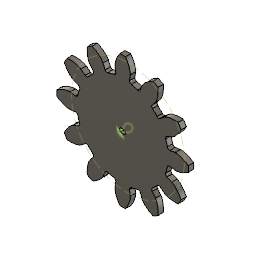
new wheel (Autodesk Fusion 360 design; units mm, degrees)
description: Spur Gear; Module: 8.7; Num Teeth: 12; Pressure Angle: 20.0; Backlash: 0.00 mm
part number: 2026-03-19-09-10-25-841
Autodesk Fusion 360 part; units mm, degrees
sketch "Base Circle" plane through (0, 0, 0) normal (0, 0, 1) x (1, 0, 0)
  circle A0 centre (0, 0) radius 42.1341
  circle A1 centre (0, 0) radius 2.7
extrude "Extrude1" add sketch "Base Circle" along normal blind 10
sketch "Gear Tooth" plane through (0, 0, 0) normal (0, 0, 1) x (1, 0, 0)
  spline S0 degree 5 poles (48.5315, -7.1267) (48.5668, -7.1319) (48.6376, -7.1411) (48.744, -7.1515) (48.8864, -7.1588) (49.065, -7.1591) (49.244, -7.153) (49.4234, -7.1431) (49.6029, -7.1312) (49.7824, -7.1179) (49.9621, -7.1029) (50.1417, -7.0859) (50.3215, -7.066) (50.5014, -7.043) (50.6813, -7.0169) (50.8612, -6.9878) (51.0412, -6.9564) (51.2211, -6.9229) (51.401, -6.8877) (51.5808, -6.8507) (51.7605, -6.812) (51.9402, -6.7714) (52.1198, -6.7289) (52.2993, -6.6844) (52.4787, -6.638) (52.658, -6.5897) (52.8372, -6.5396) (53.0163, -6.4879) (53.1952, -6.4346) (53.374, -6.3796) (53.5526, -6.3231) (53.7311, -6.265) (53.9094, -6.2053) (54.0875, -6.144) (54.2655, -6.0812) (54.4433, -6.0168) (54.6209, -5.951) (54.7983, -5.8837) (54.9754, -5.8149) (55.1524, -5.7447) (55.3292, -5.673) (55.5057, -5.6) (55.682, -5.5256) (55.8581, -5.4497) (56.0339, -5.3725) (56.2095, -5.294) (56.3849, -5.2141) (56.56, -5.1329) (56.7348, -5.0503) (56.9094, -4.9665) (57.0837, -4.8813) (57.2577, -4.7949) (57.4314, -4.7072) (57.6049, -4.6183) (57.778, -4.528) (57.9509, -4.4366) (58.1235, -4.3439) (58.2957, -4.25) (58.4677, -4.1549) (58.6393, -4.0585) (58.8106, -3.961) (58.9816, -3.8623) (59.1523, -3.7624) (59.3227, -3.6613) (59.4927, -3.5591) (59.6624, -3.4557) (59.8317, -3.3512) (60.0007, -3.2455) (60.1693, -3.1387) (60.3376, -3.0308) (60.5055, -2.9217) (60.6395, -2.8336) (60.7399, -2.767) (60.8067, -2.7224) (60.8401, -2.7) knots 0 0 0 0 0 0 0.01428571 0.02857143 0.04285714 0.05714286 0.07142857 0.08571429 0.1 0.11428571 0.12857143 0.14285714 0.15714286 0.17142857 0.18571429 0.2 0.21428571 0.22857143 0.24285714 0.25714286 0.27142857 0.28571429 0.3 0.31428571 0.32857143 0.34285714 0.35714286 0.37142857 0.38571429 0.4 0.41428571 0.42857143 0.44285714 0.45714286 0.47142857 0.48571429 0.5 0.51428571 0.52857143 0.54285714 0.55714286 0.57142857 0.58571429 0.6 0.61428571 0.62857143 0.64285714 0.65714286 0.67142857 0.68571429 0.7 0.71428571 0.72857143 0.74285714 0.75714286 0.77142857 0.78571429 0.8 0.81428571 0.82857143 0.84285714 0.85714286 0.87142857 0.88571429 0.9 0.91428571 0.92857143 0.94285714 0.95714286 0.97142857 0.98571429 1 1 1 1 1 1
  spline S1 degree 5 poles (48.5315, 7.1267) (48.5668, 7.1319) (48.6376, 7.1411) (48.744, 7.1515) (48.8864, 7.1588) (49.065, 7.1591) (49.244, 7.153) (49.4234, 7.1431) (49.6029, 7.1312) (49.7824, 7.1179) (49.9621, 7.1029) (50.1417, 7.0859) (50.3215, 7.066) (50.5014, 7.043) (50.6813, 7.0169) (50.8612, 6.9878) (51.0412, 6.9564) (51.2211, 6.9229) (51.401, 6.8877) (51.5808, 6.8507) (51.7605, 6.812) (51.9402, 6.7714) (52.1198, 6.7289) (52.2993, 6.6844) (52.4787, 6.638) (52.658, 6.5897) (52.8372, 6.5396) (53.0163, 6.4879) (53.1952, 6.4346) (53.374, 6.3796) (53.5526, 6.3231) (53.7311, 6.265) (53.9094, 6.2053) (54.0875, 6.144) (54.2655, 6.0812) (54.4433, 6.0168) (54.6209, 5.951) (54.7983, 5.8837) (54.9754, 5.8149) (55.1524, 5.7447) (55.3292, 5.673) (55.5057, 5.6) (55.682, 5.5256) (55.8581, 5.4497) (56.0339, 5.3725) (56.2095, 5.294) (56.3849, 5.2141) (56.56, 5.1329) (56.7348, 5.0503) (56.9094, 4.9665) (57.0837, 4.8813) (57.2577, 4.7949) (57.4314, 4.7072) (57.6049, 4.6183) (57.778, 4.528) (57.9509, 4.4366) (58.1235, 4.3439) (58.2957, 4.25) (58.4677, 4.1549) (58.6393, 4.0585) (58.8106, 3.961) (58.9816, 3.8623) (59.1523, 3.7624) (59.3227, 3.6613) (59.4927, 3.5591) (59.6624, 3.4557) (59.8317, 3.3512) (60.0007, 3.2455) (60.1693, 3.1387) (60.3376, 3.0308) (60.5055, 2.9217) (60.6395, 2.8336) (60.7399, 2.767) (60.8067, 2.7224) (60.8401, 2.7) knots 0 0 0 0 0 0 0.01428571 0.02857143 0.04285714 0.05714286 0.07142857 0.08571429 0.1 0.11428571 0.12857143 0.14285714 0.15714286 0.17142857 0.18571429 0.2 0.21428571 0.22857143 0.24285714 0.25714286 0.27142857 0.28571429 0.3 0.31428571 0.32857143 0.34285714 0.35714286 0.37142857 0.38571429 0.4 0.41428571 0.42857143 0.44285714 0.45714286 0.47142857 0.48571429 0.5 0.51428571 0.52857143 0.54285714 0.55714286 0.57142857 0.58571429 0.6 0.61428571 0.62857143 0.64285714 0.65714286 0.67142857 0.68571429 0.7 0.71428571 0.72857143 0.74285714 0.75714286 0.77142857 0.78571429 0.8 0.81428571 0.82857143 0.84285714 0.85714286 0.87142857 0.88571429 0.9 0.91428571 0.92857143 0.94285714 0.95714286 0.97142857 0.98571429 1 1 1 1 1 1
  arc A0 (60.8401, -2.7) -> (60.8401, 2.7) centre (0, 0) ccw
  line L0 (41.6771, -6.1201) -> (48.5315, -7.1267)
  line L1 (41.6771, 6.1201) -> (48.5315, 7.1267)
  line L2 (41.6771, -6.1201) -> (41.6771, 6.1201)
  point P0 (49.3841, -7.1449)
  point P1 (50.2491, -7.0736)
  point P2 (51.1217, -6.9412)
  point P3 (51.9999, -6.757)
  point P4 (52.8822, -6.5264)
  point P5 (53.7674, -6.2526)
  point P6 (54.6544, -5.938)
  point P7 (55.5422, -5.5843)
  point P8 (56.4301, -5.1929)
  point P9 (57.3171, -4.7647)
  point P10 (58.2025, -4.3007)
  point P11 (59.0853, -3.8015)
  point P12 (59.9647, -3.2678)
  point P13 (49.3841, 7.1449)
  point P14 (50.2491, 7.0736)
  point P15 (51.1217, 6.9412)
  point P16 (51.9999, 6.757)
  point P17 (52.8822, 6.5264)
  point P18 (53.7674, 6.2526)
  point P19 (54.6544, 5.938)
  point P20 (55.5422, 5.5843)
  point P21 (56.4301, 5.1929)
  point P22 (57.3171, 4.7647)
  point P23 (58.2025, 4.3007)
  point P24 (59.0853, 3.8015)
  point P25 (59.9647, 3.2678)
extrude "Extrude2" add sketch "Gear Tooth" along normal blind 10
fillet "Fillet1" radius 2 2 edges at (41.687, -6.1216, 5) (41.687, 6.1216, 5)
pattern_circular "C-Pattern1" count 12 over 360 about axis through (0, 0, 0) along (0, 0, 1) of "Extrude2", "Fillet1"
sketch "Diametrial Pitch Circle" plane through (0, 0, 0) normal (0, 0, 1) x (1, 0, 0)
  circle A0 centre (0, 0) radius 52.2 construction
extrude "Extrude3" cut 1 faces at (24.7473, -14.2102, 10) along direction (0, 0, -1) blind 5
sketch "Sketch4" plane through (0, 0, 5) normal (0, 0, 1) x (1, 0, 0)
  arc A0 (39.8269, -13.7514) -> (41.3668, -8.0044) centre (0, 0) ccw
  arc A1 (43.621, -6.4056) -> (41.3668, -8.0044) centre (43.3304, -8.3843) ccw
  line L0 (43.621, -6.4056) -> (48.5315, -7.1267)
  spline S0 degree 3 poles (60.8401, -2.7) (59.1145, -3.8556) (57.2554, -4.8835) (52.319, -6.9059) (50.289, -7.0824) (49.1033, -7.1662) (48.8143, -7.1682) (48.5315, -7.1267) knots -0.2727 -0.2727 -0.2727 -0.2727 -0.199923 -0.199923 -0.085763 -0.085763 0 0 0 0
  arc A2 (60.8401, -2.7) -> (60.8401, 2.7) centre (0, 0) ccw
  spline S1 degree 3 poles (48.5315, 7.1267) (49.4623, 7.2633) (51.1328, 6.9471) (52.3261, 6.6899) (53.3852, 6.4257) (56.9135, 5.0713) (58.958, 3.9603) (60.8401, 2.7) knots -1.50599 -1.50599 -1.50599 -1.50599 -1.133496 -1.133496 -0.679542 -0.679542 0 0 0 0
  line L1 (48.5315, 7.1267) -> (43.621, 6.4056)
  arc A3 (41.3668, 8.0044) -> (43.621, 6.4056) centre (43.3304, 8.3843) ccw
  arc A4 (41.3668, 8.0044) -> (39.8269, 13.7514) centre (0, 0) ccw
  arc A5 (40.9796, 16.2631) -> (39.8269, 13.7514) centre (41.7174, 14.4041) ccw
  line L2 (40.9796, 16.2631) -> (45.5928, 18.0939)
  spline S2 degree 3 poles (54.0391, 28.0818) (53.1224, 26.2182) (52.0264, 24.3984) (48.7626, 20.1788) (47.0927, 19.011) (46.1078, 18.3456) (45.8585, 18.1993) (45.5928, 18.0939) knots -0.2727 -0.2727 -0.2727 -0.2727 -0.199923 -0.199923 -0.085763 -0.085763 0 0 0 0
  arc A6 (54.0391, 28.0818) -> (51.3391, 32.7583) centre (0, 0) ccw
  spline S3 degree 3 poles (38.4662, 30.4376) (39.2039, 31.0214) (40.8087, 31.5827) (41.9708, 31.9566) (43.0201, 32.2574) (46.7528, 32.8486) (49.0789, 32.9087) (51.3391, 32.7583) knots -1.50599 -1.50599 -1.50599 -1.50599 -1.133496 -1.133496 -0.679542 -0.679542 0 0 0 0
  line L3 (38.4662, 30.4376) -> (34.5741, 27.3579)
  arc A7 (31.8225, 27.6154) -> (34.5741, 27.3579) centre (33.333, 28.9262) ccw
  arc A8 (31.8225, 27.6154) -> (27.6154, 31.8225) centre (0, 0) ccw
  arc A9 (27.3579, 34.5741) -> (27.6154, 31.8225) centre (28.9262, 33.333) ccw
  line L4 (27.3579, 34.5741) -> (30.4376, 38.4662)
  spline S4 degree 3 poles (32.7583, 51.3391) (32.8962, 49.2668) (32.8569, 47.1428) (32.1402, 41.8567) (31.278, 40.0104) (30.7577, 38.9416) (30.615, 38.6903) (30.4376, 38.4662) knots -0.2727 -0.2727 -0.2727 -0.2727 -0.199923 -0.199923 -0.085763 -0.085763 0 0 0 0
  arc A10 (32.7583, 51.3391) -> (28.0818, 54.0391) centre (0, 0) ccw
  spline S5 degree 3 poles (18.0939, 45.5928) (18.4409, 46.4673) (19.5501, 47.7558) (20.3695, 48.6607) (21.1278, 49.4457) (24.0648, 51.8242) (26.0492, 53.0393) (28.0818, 54.0391) knots -1.50599 -1.50599 -1.50599 -1.50599 -1.133496 -1.133496 -0.679542 -0.679542 0 0 0 0
  line L5 (18.0939, 45.5928) -> (16.2631, 40.9796)
  arc A11 (13.7514, 39.8269) -> (16.2631, 40.9796) centre (14.4041, 41.7174) ccw
  arc A12 (13.7514, 39.8269) -> (8.0044, 41.3668) centre (0, 0) ccw
  arc A13 (6.4056, 43.621) -> (8.0044, 41.3668) centre (8.3843, 43.3304) ccw
  line L6 (6.4056, 43.621) -> (7.1267, 48.5315)
  spline S6 degree 3 poles (2.7, 60.8401) (3.8556, 59.1145) (4.8835, 57.2554) (6.9059, 52.319) (7.0824, 50.289) (7.1662, 49.1033) (7.1682, 48.8143) (7.1267, 48.5315) knots -0.2727 -0.2727 -0.2727 -0.2727 -0.199923 -0.199923 -0.085763 -0.085763 0 0 0 0
  arc A14 (2.7, 60.8401) -> (-2.7, 60.8401) centre (0, 0) ccw
  spline S7 degree 3 poles (-7.1267, 48.5315) (-7.2633, 49.4623) (-6.9471, 51.1328) (-6.6899, 52.3261) (-6.4257, 53.3852) (-5.0713, 56.9135) (-3.9603, 58.958) (-2.7, 60.8401) knots -1.50599 -1.50599 -1.50599 -1.50599 -1.133496 -1.133496 -0.679542 -0.679542 0 0 0 0
  line L7 (-7.1267, 48.5315) -> (-6.4056, 43.621)
  arc A15 (-8.0044, 41.3668) -> (-6.4056, 43.621) centre (-8.3843, 43.3304) ccw
  arc A16 (-8.0044, 41.3668) -> (-13.7514, 39.8269) centre (0, 0) ccw
  arc A17 (-16.2631, 40.9796) -> (-13.7514, 39.8269) centre (-14.4041, 41.7174) ccw
  line L8 (-16.2631, 40.9796) -> (-18.0939, 45.5928)
  spline S8 degree 3 poles (-28.0818, 54.0391) (-26.2182, 53.1224) (-24.3984, 52.0264) (-20.1788, 48.7626) (-19.011, 47.0927) (-18.3456, 46.1078) (-18.1993, 45.8585) (-18.0939, 45.5928) knots -0.2727 -0.2727 -0.2727 -0.2727 -0.199923 -0.199923 -0.085763 -0.085763 0 0 0 0
  arc A18 (-28.0818, 54.0391) -> (-32.7583, 51.3391) centre (0, 0) ccw
  spline S9 degree 3 poles (-30.4376, 38.4662) (-31.0214, 39.2039) (-31.5827, 40.8087) (-31.9566, 41.9708) (-32.2574, 43.0201) (-32.8486, 46.7528) (-32.9087, 49.0789) (-32.7583, 51.3391) knots -1.50599 -1.50599 -1.50599 -1.50599 -1.133496 -1.133496 -0.679542 -0.679542 0 0 0 0
  line L9 (-30.4376, 38.4662) -> (-27.3579, 34.5741)
  arc A19 (-27.6154, 31.8225) -> (-27.3579, 34.5741) centre (-28.9262, 33.333) ccw
  arc A20 (-27.6154, 31.8225) -> (-31.8225, 27.6154) centre (0, 0) ccw
  arc A21 (-34.5741, 27.3579) -> (-31.8225, 27.6154) centre (-33.333, 28.9262) ccw
  line L10 (-34.5741, 27.3579) -> (-38.4662, 30.4376)
  spline S10 degree 3 poles (-51.3391, 32.7583) (-49.2668, 32.8962) (-47.1428, 32.8569) (-41.8567, 32.1402) (-40.0104, 31.278) (-38.9416, 30.7577) (-38.6903, 30.615) (-38.4662, 30.4376) knots -0.2727 -0.2727 -0.2727 -0.2727 -0.199923 -0.199923 -0.085763 -0.085763 0 0 0 0
  arc A22 (-51.3391, 32.7583) -> (-54.0391, 28.0818) centre (0, 0) ccw
  spline S11 degree 3 poles (-45.5928, 18.0939) (-46.4673, 18.4409) (-47.7558, 19.5501) (-48.6607, 20.3695) (-49.4457, 21.1278) (-51.8242, 24.0648) (-53.0393, 26.0492) (-54.0391, 28.0818) knots -1.50599 -1.50599 -1.50599 -1.50599 -1.133496 -1.133496 -0.679542 -0.679542 0 0 0 0
  line L11 (-45.5928, 18.0939) -> (-40.9796, 16.2631)
  arc A23 (-39.8269, 13.7514) -> (-40.9796, 16.2631) centre (-41.7174, 14.4041) ccw
  arc A24 (-39.8269, 13.7514) -> (-41.3668, 8.0044) centre (0, 0) ccw
  arc A25 (-43.621, 6.4056) -> (-41.3668, 8.0044) centre (-43.3304, 8.3843) ccw
  line L12 (-43.621, 6.4056) -> (-48.5315, 7.1267)
  spline S12 degree 3 poles (-60.8401, 2.7) (-59.1145, 3.8556) (-57.2554, 4.8835) (-52.319, 6.9059) (-50.289, 7.0824) (-49.1033, 7.1662) (-48.8143, 7.1682) (-48.5315, 7.1267) knots -0.2727 -0.2727 -0.2727 -0.2727 -0.199923 -0.199923 -0.085763 -0.085763 0 0 0 0
  arc A26 (-60.8401, 2.7) -> (-60.8401, -2.7) centre (0, 0) ccw
  spline S13 degree 3 poles (-48.5315, -7.1267) (-49.4623, -7.2633) (-51.1328, -6.9471) (-52.3261, -6.6899) (-53.3852, -6.4257) (-56.9135, -5.0713) (-58.958, -3.9603) (-60.8401, -2.7) knots -1.50599 -1.50599 -1.50599 -1.50599 -1.133496 -1.133496 -0.679542 -0.679542 0 0 0 0
  line L13 (-48.5315, -7.1267) -> (-43.621, -6.4056)
  arc A27 (-41.3668, -8.0044) -> (-43.621, -6.4056) centre (-43.3304, -8.3843) ccw
  arc A28 (-41.3668, -8.0044) -> (-39.8269, -13.7514) centre (0, 0) ccw
  arc A29 (-40.9796, -16.2631) -> (-39.8269, -13.7514) centre (-41.7174, -14.4041) ccw
  line L14 (-40.9796, -16.2631) -> (-45.5928, -18.0939)
  spline S14 degree 3 poles (-54.0391, -28.0818) (-53.1224, -26.2182) (-52.0264, -24.3984) (-48.7626, -20.1788) (-47.0927, -19.011) (-46.1078, -18.3456) (-45.8585, -18.1993) (-45.5928, -18.0939) knots -0.2727 -0.2727 -0.2727 -0.2727 -0.199923 -0.199923 -0.085763 -0.085763 0 0 0 0
  arc A30 (-54.0391, -28.0818) -> (-51.3391, -32.7583) centre (0, 0) ccw
  spline S15 degree 3 poles (-38.4662, -30.4376) (-39.2039, -31.0214) (-40.8087, -31.5827) (-41.9708, -31.9566) (-43.0201, -32.2574) (-46.7528, -32.8486) (-49.0789, -32.9087) (-51.3391, -32.7583) knots -1.50599 -1.50599 -1.50599 -1.50599 -1.133496 -1.133496 -0.679542 -0.679542 0 0 0 0
  line L15 (-38.4662, -30.4376) -> (-34.5741, -27.3579)
  arc A31 (-31.8225, -27.6154) -> (-34.5741, -27.3579) centre (-33.333, -28.9262) ccw
  arc A32 (-31.8225, -27.6154) -> (-27.6154, -31.8225) centre (0, 0) ccw
  arc A33 (-27.3579, -34.5741) -> (-27.6154, -31.8225) centre (-28.9262, -33.333) ccw
  line L16 (-27.3579, -34.5741) -> (-30.4376, -38.4662)
  spline S16 degree 3 poles (-32.7583, -51.3391) (-32.8962, -49.2668) (-32.8569, -47.1428) (-32.1402, -41.8567) (-31.278, -40.0104) (-30.7577, -38.9416) (-30.615, -38.6903) (-30.4376, -38.4662) knots -0.2727 -0.2727 -0.2727 -0.2727 -0.199923 -0.199923 -0.085763 -0.085763 0 0 0 0
  arc A34 (-32.7583, -51.3391) -> (-28.0818, -54.0391) centre (0, 0) ccw
  spline S17 degree 3 poles (-18.0939, -45.5928) (-18.4409, -46.4673) (-19.5501, -47.7558) (-20.3695, -48.6607) (-21.1278, -49.4457) (-24.0648, -51.8242) (-26.0492, -53.0393) (-28.0818, -54.0391) knots -1.50599 -1.50599 -1.50599 -1.50599 -1.133496 -1.133496 -0.679542 -0.679542 0 0 0 0
  line L17 (-18.0939, -45.5928) -> (-16.2631, -40.9796)
  arc A35 (-13.7514, -39.8269) -> (-16.2631, -40.9796) centre (-14.4041, -41.7174) ccw
  arc A36 (-13.7514, -39.8269) -> (-8.0044, -41.3668) centre (0, 0) ccw
  arc A37 (-6.4056, -43.621) -> (-8.0044, -41.3668) centre (-8.3843, -43.3304) ccw
  line L18 (-6.4056, -43.621) -> (-7.1267, -48.5315)
  spline S18 degree 3 poles (-2.7, -60.8401) (-3.8556, -59.1145) (-4.8835, -57.2554) (-6.9059, -52.319) (-7.0824, -50.289) (-7.1662, -49.1033) (-7.1682, -48.8143) (-7.1267, -48.5315) knots -0.2727 -0.2727 -0.2727 -0.2727 -0.199923 -0.199923 -0.085763 -0.085763 0 0 0 0
  arc A38 (-2.7, -60.8401) -> (2.7, -60.8401) centre (0, 0) ccw
  spline S19 degree 3 poles (7.1267, -48.5315) (7.2633, -49.4623) (6.9471, -51.1328) (6.6899, -52.3261) (6.4257, -53.3852) (5.0713, -56.9135) (3.9603, -58.958) (2.7, -60.8401) knots -1.50599 -1.50599 -1.50599 -1.50599 -1.133496 -1.133496 -0.679542 -0.679542 0 0 0 0
  line L19 (7.1267, -48.5315) -> (6.4056, -43.621)
  arc A39 (8.0044, -41.3668) -> (6.4056, -43.621) centre (8.3843, -43.3304) ccw
  arc A40 (8.0044, -41.3668) -> (13.7514, -39.8269) centre (0, 0) ccw
  arc A41 (16.2631, -40.9796) -> (13.7514, -39.8269) centre (14.4041, -41.7174) ccw
  line L20 (16.2631, -40.9796) -> (18.0939, -45.5928)
  spline S20 degree 3 poles (28.0818, -54.0391) (26.2182, -53.1224) (24.3984, -52.0264) (20.1788, -48.7626) (19.011, -47.0927) (18.3456, -46.1078) (18.1993, -45.8585) (18.0939, -45.5928) knots -0.2727 -0.2727 -0.2727 -0.2727 -0.199923 -0.199923 -0.085763 -0.085763 0 0 0 0
  arc A42 (28.0818, -54.0391) -> (32.7583, -51.3391) centre (0, 0) ccw
  spline S21 degree 3 poles (30.4376, -38.4662) (31.0214, -39.2039) (31.5827, -40.8087) (31.9566, -41.9708) (32.2574, -43.0201) (32.8486, -46.7528) (32.9087, -49.0789) (32.7583, -51.3391) knots -1.50599 -1.50599 -1.50599 -1.50599 -1.133496 -1.133496 -0.679542 -0.679542 0 0 0 0
  line L21 (30.4376, -38.4662) -> (27.3579, -34.5741)
  arc A43 (27.6154, -31.8225) -> (27.3579, -34.5741) centre (28.9262, -33.333) ccw
  arc A44 (27.6154, -31.8225) -> (31.8225, -27.6154) centre (0, 0) ccw
  arc A45 (34.5741, -27.3579) -> (31.8225, -27.6154) centre (33.333, -28.9262) ccw
  line L22 (34.5741, -27.3579) -> (38.4662, -30.4376)
  spline S22 degree 3 poles (51.3391, -32.7583) (49.2668, -32.8962) (47.1428, -32.8569) (41.8567, -32.1402) (40.0104, -31.278) (38.9416, -30.7577) (38.6903, -30.615) (38.4662, -30.4376) knots -0.2727 -0.2727 -0.2727 -0.2727 -0.199923 -0.199923 -0.085763 -0.085763 0 0 0 0
  arc A46 (51.3391, -32.7583) -> (54.0391, -28.0818) centre (0, 0) ccw
  spline S23 degree 3 poles (45.5928, -18.0939) (46.4673, -18.4409) (47.7558, -19.5501) (48.6607, -20.3695) (49.4457, -21.1278) (51.8242, -24.0648) (53.0393, -26.0492) (54.0391, -28.0818) knots -1.50599 -1.50599 -1.50599 -1.50599 -1.133496 -1.133496 -0.679542 -0.679542 0 0 0 0
  line L23 (45.5928, -18.0939) -> (40.9796, -16.2631)
  arc A47 (39.8269, -13.7514) -> (40.9796, -16.2631) centre (41.7174, -14.4041) ccw
  circle A48 centre (0, 0) radius 2.7
  circle A49 centre (0, 0) radius 2.7
  line L24 (0, 0) -> (0, -1.85)
  line L25 (0, -1.85) -> (-1.9666, -1.85)
  line L26 (0, -1.85) -> (1.9666, -1.85)
  line L27 (1.9666, -1.85) -> (1.9666, 1.85)
  line L28 (1.9666, 1.85) -> (-1.9666, 1.85)
  line L29 (-1.9666, -1.85) -> (-1.9666, 1.85)
  dimension "d11" = 1.85
  constraint coincident A0.centre A2.centre
  constraint vertical L24
  constraint coincident A48 L25.end
  constraint perpendicular L24 L25
  constraint coincident A48 L26.end
  constraint perpendicular L24 L26
  constraint coincident A49 L27.end
  constraint perpendicular L26 L27
  constraint coincident A49 L28.end
  constraint perpendicular L27 L28
  measures "d11" distance of A0.centre L24.end
extrude "Extrude4" add sketch "Sketch4" against normal blind 5 contours A48 A49 L28 | A48 A49 L25 L26
sketch "Sketch5" plane through (0, 0, 0) normal (0, 0, 1) x (1, 0, 0)
  circle A0 centre (0, 0) radius 7.5
  dimension "d14" = 15
  constraint coincident A0.centre origin
  measures "d14" diameter of A0
extrude "Extrude5" add sketch "Sketch5" against normal blind 5
extrude "Extrude6" cut 1 faces at (-0.7337, 0.7122, 0) along direction (0, 0, -1) blind 21
fillet "Fillet2" radius 112 1 edges at (-6.9925, -2.7121, 0)
fillet "Fillet3" radius 5 1 edges at (-6.9925, 2.7121, -5)
named bodies: "Spur Gear (12 teeth)"
